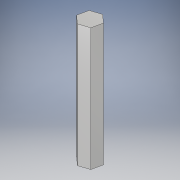
# Autodesk Inventor part: Dex shaft
Saved by Autodesk Inventor 2018 (Build 220112000, 112)
## iProperties
Created: 2018-03-20
Part Number: Dex shaft
Material: Generic
Document SubType Name: Modeling
Designer: prakh
Density: 1 g/cm^3
Appearance: Aluminum - Dark
Author: prakh
Autodesk Inventor part; units mm, degrees
ref_plane "YZ Plane" through (0, 0, 0) normal (1, 0, 0) x (0, 1, 0)
ref_plane "XZ Plane" through (0, 0, 0) normal (0, 1, 0) x (-1, 0, 0)
ref_plane "XY Plane" through (0, 0, 0) normal (0, 0, 1) x (1, 0, 0)
sketch "Sketch1" plane through (0, 0, 0) normal (0, 1, 0) x (-1, 0, 0)
  line L0 (1.1628, 5.3749) -> (5.2362, 1.6804)
  line L1 (5.2362, 1.6804) -> (4.0734, -3.6945)
  line L2 (4.0734, -3.6945) -> (-1.1628, -5.3749)
  line L3 (-1.1628, -5.3749) -> (-5.2362, -1.6804)
  line L4 (-5.2362, -1.6804) -> (-4.0734, 3.6945)
  line L5 (-4.0734, 3.6945) -> (1.1628, 5.3749)
  point P0 (0, 0)
  point P1 (0, 0)
  dimension "d0" = 9.525
  constraints: 12 end point, 1 coincident, 13 other
  measures "d0" distance between parallel lines of L3 L0
extrude "Extrusion1" add sketch "Sketch1" along normal blind 63.5
body "Solid1"
